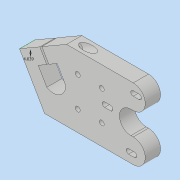
# Autodesk Inventor part: MMplate1
Saved by Autodesk Inventor 2017 (Build 210142000, 142)
## iProperties
Created: 2016-12-19
Part Number: MMplate1
Material: Generic
Document SubType Name: Modeling
Designer: Joshua Yuan
Density: 1 g/cm^3
Appearance: Default
Author: Joshua Yuan
Autodesk Inventor part; units mm, degrees
ref_plane "YZ Plane" through (0, 0, 0) normal (1, 0, 0) x (0, 1, 0)
ref_plane "XZ Plane" through (0, 0, 0) normal (0, 1, 0) x (-1, 0, 0)
ref_plane "XY Plane" through (0, 0, 0) normal (0, 0, 1) x (1, 0, 0)
sketch "Sketch1" plane through (0, 0, 0) normal (0, 0, 1) x (1, 0, 0)
  line L0 (31.4659, 48.2287) -> (38.5187, 52.3007)
  line L1 (47.2721, 57.4272) -> (54.3841, 45.1089)
  line L2 (31.4659, 48.2287) -> (38.5779, 35.9104)
  arc A0 (38.5779, 35.9104) -> (54.3841, 45.1089) centre (43.9742, 44.8171) ccw
  line L3 (15.8522, 52.4124) -> (32.8037, 62.1993)
  line L4 (15.8522, 52.4124) -> (36.8033, 16.1239)
  line L5 (-9.2352, 0) -> (166.3765, 0) projected
  line L6 (0, -0.1512) -> (0, 91.432) projected
  line L7 (34.5043, 63.2539) -> (40.2193, 53.3553)
  line L8 (32.8037, 62.1993) -> (38.5187, 52.3007)
  line L9 (34.5043, 63.2539) -> (55.0637, 75.1239)
  line L10 (40.2193, 53.3553) -> (47.2721, 57.4272)
  arc A1 (113.3788, 16.5188) -> (110.5982, 16.1938) centre (108.5682, 45.6239) ccw
  circle A2 centre (43.5282, 45.6239) radius 3.975 construction
  circle A3 centre (64.3841, 33.1239) radius 2.0193
  circle A4 centre (84.3841, 33.1239) radius 2.0193
  circle A5 centre (64.3841, 58.1239) radius 2.0193
  circle A6 centre (84.3841, 58.1239) radius 2.0193
  arc A7 (111.394, 54.7201) -> (118.0707, 44.9701) centre (108.5682, 45.6239) ccw
  circle A8 centre (86.7313, 47.5344) radius 2
  circle A9 centre (110.4787, 67.4608) radius 2
  circle A10 centre (130.4051, 43.7134) radius 2
  circle A11 centre (106.6577, 23.787) radius 2
  line L11 (110.4787, 67.4608) -> (106.6577, 23.787) construction
  line L12 (130.4051, 43.7134) -> (86.7313, 47.5344) construction
  circle A12 centre (91.7313, 47.5344) radius 2
  circle A13 centre (115.4787, 67.4608) radius 2
  circle A14 centre (111.6577, 23.787) radius 2
  circle A15 centre (135.4051, 43.7134) radius 2
  circle A16 centre (110.5982, 45.6239) radius 29.5 construction
  circle A17 centre (110.5982, 45.6239) radius 9.525 construction
  line L13 (115.4787, 69.4608) -> (110.4787, 69.4608)
  line L14 (110.4787, 65.4608) -> (115.4787, 65.4608)
  line L15 (106.6577, 25.787) -> (111.6577, 25.787)
  line L16 (111.6577, 21.787) -> (106.6577, 21.787)
  line L17 (86.7313, 49.5344) -> (91.7313, 49.5344)
  line L18 (91.7313, 45.5344) -> (86.7313, 45.5344)
  line L19 (110.5982, 45.6239) -> (43.5282, 45.6239) construction
  circle A18 centre (88.7613, 47.5344) radius 2 construction
  circle A19 centre (112.5087, 67.4608) radius 2 construction
  circle A20 centre (132.4351, 43.7134) radius 2 construction
  circle A21 centre (108.6877, 23.787) radius 2 construction
  line L20 (130.4051, 45.7134) -> (135.4051, 45.7134)
  line L21 (135.4051, 41.7134) -> (130.4051, 41.7134)
  line L22 (132.4351, 43.7134) -> (88.7613, 47.5344) construction
  line L23 (112.5087, 67.4608) -> (108.6877, 23.787) construction
  line L24 (64.3841, 58.1239) -> (64.3841, 33.1239) construction
  line L25 (84.3841, 33.1239) -> (84.3841, 58.1239) construction
  arc A22 (110.5982, 55.1489) -> (110.5982, 75.1239) centre (110.5982, 65.1364) ccw
  arc A23 (110.5982, 16.1239) -> (110.5982, 36.0989) centre (110.5982, 26.1114) ccw
  line L26 (110.5982, 16.1239) -> (110.5982, 75.1239) construction
  line L27 (110.5982, 36.0989) -> (108.5682, 36.0989)
  line L28 (110.5982, 55.1489) -> (108.5682, 55.1489)
  arc A24 (118.0707, 44.9701) -> (111.394, 54.7201) centre (108.5682, 45.6239) ccw construction
  line L29 (108.5682, 16.1239) -> (36.8033, 16.1239)
  line L30 (55.0637, 75.1239) -> (110.5982, 75.1239)
  line L31 (110.5982, 16.1239) -> (108.5682, 16.1239)
  point P0 (114.9222, 74.4315)
  point P1 (112.9787, 65.4608)
  point P2 (108.5682, 45.6239)
  dimension "d8" = 18.288
  dimension "d9" = 14.224
  dimension "d10" = 10.414
  dimension "d13" = 11.43
  dimension "d14" = 11.43
  dimension "d15" = 2
  dimension "d17" = 59
  dimension "d18" = 7.95
  dimension "d19" = 9.144
  dimension "d20" = 9.2717
  dimension "d21" = 30
  dimension "d22" = 8.35
  dimension "d23" = 65.04
  dimension "d25" = 4.0386
  dimension "d26" = 4.0386
  dimension "d27" = 4.0386
  dimension "d28" = 4.0386
  dimension "d32" = 19.05
  dimension "d33" = 4
  dimension "d34" = 4
  dimension "d35" = 4
  dimension "d36" = 4
  dimension "d38" = 31
  dimension "d39" = 31
  dimension "d40" = 31
  dimension "d41" = 31
  dimension "d42" = 20
  dimension "d43" = 25
  dimension "d44" = 25
  dimension "d46" = 10
  dimension "d49" = 4
  dimension "d50" = 4
  dimension "d51" = 4
  dimension "d52" = 4
  dimension "d53" = 5
  dimension "d54" = 59
  dimension "d55" = 67.07
  dimension "d56" = 19.05
  dimension "d57" = 5
  dimension "d58" = 5
  dimension "d59" = 5
  dimension "d60" = 4
  dimension "d61" = 4
  dimension "d62" = 4
  dimension "d63" = 4
  dimension "d68" = 5
  dimension "d69" = 5
  dimension "d70" = 31
  dimension "d71" = 31
  dimension "d72" = 31
  dimension "d73" = 31
  constraints: 60 end point, 37 point on circle, 25 centre point, 18 tangent, 12 horizontal, 8 midpoint, 8 perpendicular, 7 point on line, 5 equal length, 5 parallel, 3 coincident, 3 vertical, 2 symmetric about line
  measures "d8" distance of L0.start L1.start
  measures "d9" distance of L0.start L2.end
  measures "d10" radius of A0
  measures "d13" distance between parallel lines of L4 L2
  measures "d14" distance of L7.start L7.end
  measures "d15" distance between parallel lines of L8 L7
  measures "d17" diameter of A1
  measures "d18" diameter of A2
  measures "d19" distance from line of L1 L19.end
  measures "d20" distance from line of L10 A0.centre
  measures "d21" angle of L5 L0
  measures "d22" distance from line of L10 L19.end
  measures "d23" distance of L19.end A1.centre
  measures "d25" diameter of A3
  measures "d26" diameter of A6
  measures "d27" diameter of A4
  measures "d28" diameter of A5
  measures "d32" diameter of A7
  measures "d33" diameter of A8
  measures "d34" diameter of A9
  measures "d35" diameter of A10
  measures "d36" diameter of A11
  measures "d38" distance of L12.start L11.end
  measures "d39" distance of L11.start L12.start
  measures "d40" distance of A8.centre L11.end
  measures "d41" distance of A8.centre L11.start
  measures "d42" distance of L24.start L25.end
  measures "d43" distance of L24.end L24.start
  measures "d44" distance of L25.start L25.end
  measures "d46" horizontal distance of L1.end L24.start
  measures "d49" diameter of A12
  measures "d50" diameter of A13
  measures "d51" diameter of A14
  measures "d52" diameter of A15
  measures "d53" distance of A8.centre A12.centre
  measures "d54" diameter of A16
  measures "d55" distance of L19.end A16.centre
  measures "d56" diameter of A17
  measures "d57" distance of L11.end A14.centre
  measures "d58" distance of A15.centre L12.start
  measures "d59" distance of L11.start A13.centre
  measures "d60" diameter of A18
  measures "d61" diameter of A19
  measures "d62" diameter of A20
  measures "d63" diameter of A21
  measures "d68" angle of L19 L22
  measures "d69" angle of L19 L12
  measures "d70" distance of L22.start L23.start
  measures "d71" distance of L23.end L22.start
  measures "d72" distance of L23.end L22.end
  measures "d73" distance of L22.end L23.start
extrude "Extrusion7" add sketch "Sketch1" along normal blind 12.7 contours L2 A0 L1 L10 L7 L9 L30 A1 L29 L4 L3 L8 L0 | A1 A22 L28 A7 L27 A23 L31 | L30 A22 A1
sketch "Sketch2" plane through (36.8033, 16.1239, 0) normal (-0.8660254, -0.5, 0) x (0, 0, 1)
  line L0 (0, 30.5353) -> (12.7, 30.5353) projected
  line L1 (0, 41.9023) -> (12.7, 41.9023) projected
  line L2 (6.35, 41.9023) -> (6.35, 30.5353) construction
  circle A0 centre (6.35, 36.2188) radius 2.0193
  circle A1 centre (6.35, 36.2188) radius 3.7229
  point P0 (0, 4.438)
  dimension "d87" = 4.0386
  constraints: 3 midpoint, 2 centre point, 2 end point, 1 coincident
  measures "d87" diameter of A0
extrude "Extrusion8" cut sketch "Sketch2" against normal through all contours A0
ref_plane "Work Plane1" through (55.0637, 75.1239, 12.7) normal (-0.8660254, -0.5, 0) x (0, 0, 1)
sketch "Sketch3" plane through (55.0637, 75.1239, 12.7) normal (-0.8660254, -0.5, 0) x (0, 0, 1)
  circle A0 centre (-6.35, -5.7465) radius 2.0193 projected
  circle A1 centre (-6.35, -5.7465) radius 3.6033
  point P0 (-12.7, -37.5274)
  constraints: 1 centre point, 1 coincident
extrude "Extrusion9" cut sketch "Sketch3" against normal through all
body "Solid7"
